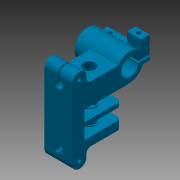
# Autodesk Inventor part: Part5
Saved by Autodesk Inventor 2015 (Build 190159000, 159)
## iProperties
Created: 2015-07-07
Part Number: Part5
Material: ABS Plastic
Document SubType Name: Modeling
Designer: eefred
Density: 1.06 g/cm^3
Appearance: Sky Blue Medium
Author: eefred
Autodesk Inventor part; units mm, degrees
ref_plane "YZ Plane" through (0, 0, 0) normal (1, 0, 0) x (0, 1, 0)
ref_plane "XZ Plane" through (0, 0, 0) normal (0, 1, 0) x (-1, 0, 0)
ref_plane "XY Plane" through (0, 0, 0) normal (0, 0, 1) x (1, 0, 0)
sketch "Sketch1" plane through (0, 0, 0) normal (1, 0, 0) x (0, 1, 0)
  line L0 (13, 5) -> (40, 5)
  line L1 (40, 5) -> (40, 20)
  line L2 (40, 20) -> (8.5, 20)
  line L3 (8.5, 20) -> (8.5, 28)
  line L4 (8.5, 28) -> (35, 28)
  line L5 (35, 28) -> (35, 31)
  line L6 (35, 31) -> (8.5, 31)
  line L7 (8.5, 31) -> (8.5, 39)
  line L8 (8.5, 39) -> (35, 39)
  line L9 (35, 39) -> (35, 45)
  line L10 (35, 45) -> (13, 45)
  circle A0 centre (5, 50) radius 1.3
  arc A1 (10, 50) -> (0, 50) centre (5, 50) ccw
  line L11 (10, 50) -> (10, 48)
  arc A2 (10, 48) -> (13, 45) centre (13, 48) ccw
  circle A3 centre (5, 0) radius 1.3
  arc A4 (0, 0) -> (10, 0) centre (5, 0) ccw
  line L12 (0, 50) -> (0, 0)
  line L13 (10, 0) -> (10, 2)
  arc A5 (13, 5) -> (10, 2) centre (13, 2) ccw
  point P0 (0, 0)
  dimension "d3" = 15
  dimension "d4" = 31.5
  dimension "d5" = 8
  dimension "d6" = 26.5
  dimension "d7" = 3
  dimension "d8" = 8
  dimension "d9" = 6
  dimension "d10" = 2.6
  dimension "d11" = 5
  dimension "d12" = 3
  dimension "d83" = 50
  dimension "d84" = 5
  dimension "d85" = 5
  dimension "d86" = 30
  dimension "d87" = 3
  constraints: 28 end point, 8 point on circle, 8 tangent, 7 perpendicular, 6 centre point, 5 vertical, 4 point on line, 2 coincident, 1 equal radius, 1 horizontal alignment, 1 vertical alignment
  measures "d3" distance of L0.end L1.end
  measures "d4" distance of L1.end L2.end
  measures "d5" distance of L2.end L3.end
  measures "d6" distance of L3.end L4.end
  measures "d7" distance of L4.end L5.end
  measures "d8" distance of L6.end L7.end
  measures "d9" distance of L8.end L9.end
  measures "d10" diameter of A0
  measures "d11" horizontal distance of point (0, 0) A0.centre
  measures "d12" radius of A2
  measures "d83" distance of A3.centre A0.centre
  measures "d84" distance from line of A3.centre L0
  measures "d85" radius of A4
  measures "d86" distance between parallel lines of L13 L1
  measures "d87" radius of A5
extrude "Extrusion5" add sketch "Sketch1" along normal blind 20
sketch "Sketch3" plane through (20, 0, 0) normal (1, 0, 0) x (0, 0, -1)
  arc A0 (-13, 50.1192) -> (-7, 50.1192) centre (-10, 41) ccw
  line L0 (0, 0) -> (0, 10)
  line L1 (-13, 50.1192) -> (-13, 55)
  line L2 (-13, 55) -> (-10.5, 55)
  line L3 (-10.5, 55) -> (-10.5, 41)
  line L4 (-10.5, 41) -> (-9.5, 41)
  line L5 (-9.5, 41) -> (-9.5, 55)
  line L6 (-9.5, 55) -> (-7, 55)
  line L7 (-7, 55) -> (-7, 50.1192)
  circle A1 centre (0, 5) radius 1.3 construction
  dimension "d21" = 9.6
  dimension "d24" = 1
  dimension "d25" = 2.5
  dimension "d26" = 2.5
  dimension "d27" = 14
  dimension "d75" = 10
  dimension "d76" = 36
  constraints: 16 end point, 4 perpendicular, 2 coincident, 2 point on circle, 2 vertical, 1 centre point, 1 horizontal, 1 midpoint, 1 point on line
  measures "d21" radius of A0
  measures "d24" distance of L3.end L4.end
  measures "d25" distance of L1.end L2.end
  measures "d26" distance of L5.end L6.end
  measures "d27" distance of L4.end L5.end
  measures "d75" horizontal distance of A1.centre A0.centre
  measures "d76" vertical distance of A1.centre A0.centre
extrude "Extrusion3" add sketch "Sketch3" against normal blind 30
sketch "Sketch11" plane through (20, 50.1192, 7) normal (0, 0, -1) x (-1, 0, 0)
  line L0 (0, 4.8808) -> (10, 4.8808)
  line L1 (10, 4.8808) -> (10, -1.2192)
  line L2 (10, -1.2192) -> (0, -1.2192)
  line L3 (0, -1.2192) -> (0, 4.8808)
  point P0 (20, -50.1192)
  dimension "d93" = 10
  dimension "d94" = 6.1
  constraints: 8 end point, 2 parallel, 1 horizontal, 1 perpendicular
  measures "d93" distance of L0.start L0.end
  measures "d94" distance of L2.end L0.start
extrude "Extrusion14" add sketch "Sketch11" along normal blind 10
sketch "Sketch4" plane through (20, 0, 0) normal (1, 0, 0) x (0, 0, -1)
  circle A0 centre (-10, 41) radius 6.2
  line L0 (-9.5, 41) -> (-10.5, 41) projected
  point P0 (0, 0)
  dimension "d30" = 12.4
  constraints: 2 coincident, 1 centre point, 1 midpoint
  measures "d30" diameter of A0
extrude "Extrusion7" cut sketch "Sketch4" against normal up to next
sketch "Sketch5" plane through (0, 0, 0) normal (0, -1, 0) x (1, 0, 0)
  circle A0 centre (10, 5) radius 3
  circle A1 centre (10, 45) radius 3
  line L0 (0, 55) -> (20, 55) construction
  line L1 (20, 50) -> (20, 0) construction
  dimension "d40" = 6
  dimension "d41" = 40
  dimension "d89" = 10
  dimension "d90" = 10
  constraints: 2 centre point, 1 equal radius, 1 vertical alignment
  measures "d40" diameter of A0
  measures "d41" distance of A1.centre A0.centre
  measures "d89" distance from line of L0 A1.centre
  measures "d90" distance from line of L1 A1.centre
extrude "Extrusion8" cut sketch "Sketch5" against normal blind 12
sketch "Sketch6" plane through (0, 0, 0) normal (0, -1, 0) x (1, 0, 0)
  line L0 (9.5, -6) -> (10.5, -6)
  line L1 (10.5, -6) -> (10.5, 3)
  line L2 (10.5, 3) -> (9.5, 3)
  line L3 (9.5, 3) -> (9.5, -6)
  line L4 (9.5, 56) -> (10.5, 56)
  line L5 (10.5, 56) -> (10.5, 47)
  line L6 (10.5, 47) -> (9.5, 47)
  line L7 (9.5, 47) -> (9.5, 56)
  line L8 (20, 58.7305) -> (20, -0.2695) construction
  circle A0 centre (10, 45) radius 3 construction
  circle A1 centre (10, 5) radius 3 construction
  point P0 (0, 0)
  point P1 (10, 3)
  point P2 (10, 47)
  dimension "d46" = 1
  dimension "d47" = 1
  dimension "d79" = 9
  dimension "d80" = 9.5
  dimension "d82" = 9
  dimension "d91" = 2
  dimension "d92" = 2
  constraints: 18 end point, 3 parallel, 2 horizontal, 2 midpoint, 2 perpendicular, 2 vertical alignment, 1 point on line
  measures "d46" distance of L0.start L0.end
  measures "d47" distance of L4.start L4.end
  measures "d79" distance of L2.end L0.start
  measures "d80" distance between parallel lines of L8 L1
  measures "d82" distance of L6.end L4.start
  measures "d91" distance of point (10, 3) A1.centre
  measures "d92" distance from line of L6 A0.centre
extrude "Extrusion9" cut sketch "Sketch6" against normal blind 12
sketch "Sketch7" plane through (20, 13, 45) normal (0, 0, 1) x (1, 0, 0)
  circle A0 centre (-10, 9) radius 4.1
  line L0 (-20, 27) -> (0, 27) projected
  line L1 (0, 22) -> (0, 0) projected
  point P0 (-20, -13)
  dimension "d53" = 8.2
  dimension "d54" = 18
  dimension "d55" = 10
  constraints: 1 centre point
  measures "d53" diameter of A0
  measures "d54" distance from line of A0.centre L0
  measures "d55" distance from line of L1 A0.centre
extrude "Extrusion10" cut sketch "Sketch7" against normal through all
sketch "Sketch8" plane through (20, 8.5, 20) normal (0, 0, 1) x (1, 0, 0)
  circle A0 centre (-10, 13.5) radius 4.1 projected
  circle A1 centre (-10, 13.5) radius 5
  point P0 (-20, -8.5)
  dimension "d58" = 10
  constraints: 1 centre point, 1 coincident
  measures "d58" diameter of A1
extrude "Extrusion11" add sketch "Sketch8" along normal blind 0.5
pattern_linear "Rectangular Pattern1" count 2 spacing 11 along (0, 0, 1) of "Extrusion11"
pattern_linear "Rectangular Pattern2" count 2 spacing 7.5 along (0, 0, 1) of "Extrusion11", "Rectangular Pattern1"
sketch "Sketch9" plane through (20, 50.1192, 7) normal (0, 0, -1) x (-1, 0, 0)
  circle A0 centre (5, 1.9308) radius 1.3
  circle A1 centre (25, 1.9308) radius 1.3
  line L0 (0, 4.8808) -> (30, 4.8808) projected
  line L1 (0, 0) -> (0, 4.8808) projected
  line L2 (30, 4.8808) -> (30, 0) projected
  point P0 (20, -50.1192)
  dimension "d67" = 2.6
  dimension "d68" = 2.95
  dimension "d69" = 5
  dimension "d70" = 5
  constraints: 2 centre point, 1 equal radius, 1 horizontal alignment
  measures "d67" diameter of A0
  measures "d68" distance from line of A0.centre L0
  measures "d69" distance from line of L1 A0.centre
  measures "d70" distance from line of L2 A1.centre
extrude "Extrusion12" cut sketch "Sketch9" along normal through all both and the other way through all
mirror "Mirror1" about plane through (0, 0, 0) normal (0, 0, 1) remove original yes
sketch "Sketch12" plane through (0, 8.5, -20) normal (0, 0, -1) x (-1, 0, 0)
  line L0 (-12.4234, 24.994) -> (-12.5505, 24.9214)
  spline S0 degree 2 poles (-12.5505, 24.9214) (-12.8047, 24.7579) (-12.9319, 24.7579) knots 0 0 0 1 1 1
  spline S1 degree 2 poles (-12.9319, 24.7579) (-13.1861, 24.7579) (-13.5493, 25.2664) (-13.5493, 25.4753) knots 0 0 0 1 2 2 2
  spline S2 degree 2 poles (-13.5493, 25.4753) (-13.5493, 25.5661) (-13.5403, 25.7114) knots 0 0 0 1 1 1
  spline S3 degree 2 poles (-13.5403, 25.7114) (-13.513, 25.8567) (-13.513, 25.893) knots 0 0 0 1 1 1
  spline S4 degree 2 poles (-13.513, 25.893) (-13.7582, 27.4276) (-13.7582, 28.0451) knots 0 0 0 1 1 1
  spline S5 degree 2 poles (-13.7582, 28.0451) (-13.7582, 29.2074) (-12.6595, 30.5604) (-11.8513, 30.5604) knots 0 0 0 1 2 2 2
  spline S6 degree 2 poles (-11.8513, 30.5604) (-11.0794, 30.5604) (-9.6901, 29.2346) (-9.2451, 28.1177) knots 0 0 0 1 2 2 2
  spline S7 degree 2 poles (-9.2451, 28.1177) (-7.7469, 29.9702) (-7.1839, 30.9327) knots 0 0 0 1 1 1
  spline S8 degree 2 poles (-7.1839, 30.9327) (-6.9841, 31.2687) (-6.6663, 31.2687) knots 0 0 0 1 1 1
  spline S9 degree 2 poles (-6.6663, 31.2687) (-6.4574, 31.2687) (-6.0397, 30.7965) (-6.0397, 30.5877) knots 0 0 0 1 2 2 2
  spline S10 degree 2 poles (-6.0397, 30.5877) (-6.0397, 30.2789) (-6.5573, 29.5161) (-7.6833, 28.1087) (-7.7923, 27.9997) knots 0 0 0 1 2 3 3 3
  spline S11 degree 2 poles (-7.7923, 27.9997) (-8.6186, 27.0099) (-8.891, 26.565) knots 0 0 0 1 1 1
  spline S12 degree 2 poles (-8.891, 26.565) (-8.891, 26.0201) (-9.4358, 26.0201) knots 0 0 0 1 1 1
  spline S13 degree 2 poles (-9.4358, 26.0201) (-9.6901, 26.0201) (-10.0624, 26.5014) (-10.0624, 26.8192) knots 0 0 0 1 2 2 2
  spline S14 degree 2 poles (-10.0624, 26.8192) (-10.0624, 26.91) (-10.0352, 27.0099) knots 0 0 0 1 1 1
  spline S15 degree 2 poles (-10.0352, 27.0099) (-10.0079, 27.1098) (-10.0079, 27.1552) knots 0 0 0 1 1 1
  spline S16 degree 2 poles (-10.0079, 27.1552) (-10.0079, 27.4821) (-11.1158, 29.2891) (-11.8513, 29.2891) knots 0 0 0 1 2 2 2
  spline S17 degree 2 poles (-11.8513, 29.2891) (-12.2145, 29.2891) (-12.7321, 28.5354) (-12.7321, 27.9452) knots 0 0 0 1 2 2 2
  spline S18 degree 2 poles (-12.7321, 27.9452) (-12.7321, 27.2551) (-12.5686, 26.4106) (-12.496, 26.3289) (-12.2417, 26.2199) (-10.3621, 25.8657) (-8.1101, 25.5752) (-7.5834, 25.5752) knots 0 0 0 1 2 3 4 5 6 6 6
  spline S19 degree 2 poles (-7.5834, 25.5752) (-7.2383, 25.5752) (-6.975, 25.6297) knots 0 0 0 1 1 1
  spline S20 degree 2 poles (-6.975, 25.6297) (-6.7026, 25.6751) (-6.5028, 25.6751) knots 0 0 0 1 1 1
  spline S21 degree 2 poles (-6.5028, 25.6751) (-6.3121, 25.6751) (-5.8853, 25.2301) (-5.8853, 24.9759) knots 0 0 0 1 2 2 2
  spline S22 degree 2 poles (-5.8853, 24.9759) (-5.8853, 24.2494) (-6.8842, 24.2494) knots 0 0 0 1 1 1
  spline S23 degree 2 poles (-6.8842, 24.2494) (-7.6924, 24.2494) (-10.6254, 24.6126) (-11.7332, 24.8578) knots 0 0 0 1 2 2 2
  spline S24 degree 2 poles (-11.7332, 24.8578) (-11.9148, 24.8941) (-12.0511, 24.9123) knots 0 0 0 1 1 1
  line L1 (-12.0511, 24.9123) -> (-12.4234, 24.994)
  point P0 (0, -8.5)
  point P1 (-13.7582, 23.5411)
  constraints: 1 other
extrude "Extrusion15" add sketch "Sketch12" along normal blind 0.5
fillet "Fillet1" radius 3 4 edges at (0, 35, -42) (0, 35, -29.5) (20, 35, -42) (20, 35, -29.5)
equation "\"d26\" = d25"
equation "\"d47\" = d46"
equation "\"d70\" = d69"
body "Solid1"
body "Solid2"
